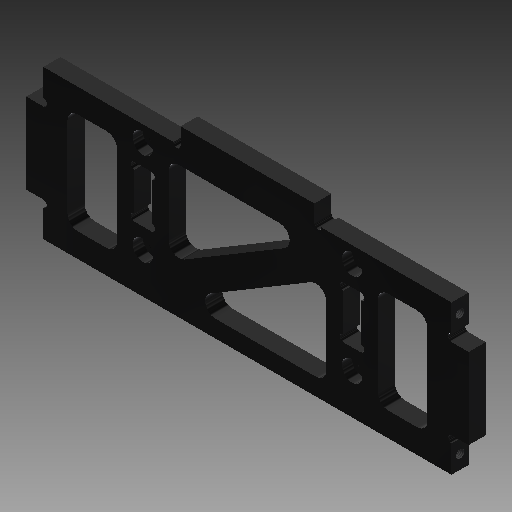
# Autodesk Inventor part: コックピット_サブフレーム_1_3
Saved by Autodesk Inventor 2018 (Build 220112000, 112)
## iProperties
Category: コックピット
Created: 2016-05-08
Part Number: コックピット_サブフレーム_1_3
Material: アセタール樹脂、黒
Document SubType Name: Modeling
Designer: hiroaki
Density: 1.425 g/cm^3
Appearance: 滑らか - 黒
Mass: 24.5118 g
Surface Area: 114.713 cm^2
Volume: 17.2013 cm^3
Author: hiroaki
Autodesk Inventor part; units mm, degrees
ref_plane "YZ Plane" through (0, 0, 0) normal (1, 0, 0) x (0, 1, 0)
ref_plane "XZ Plane" through (0, 0, 0) normal (0, 1, 0) x (-1, 0, 0)
ref_plane "XY Plane" through (0, 0, 0) normal (0, 0, 1) x (1, 0, 0)
sketch "スケッチ1" plane through (0, 0, 0) normal (0, 0, 1) x (1, 0, 0)
  line L0 (-59.5, -21.75) -> (59.5, -21.75) construction
  line L1 (59.5, -21.75) -> (59.5, 21.75) construction
  line L2 (59.5, 21.75) -> (-59.5, 21.75) construction
  line L3 (-59.5, 21.75) -> (-59.5, -21.75) construction
  line L4 (-59.5, -21.75) -> (59.5, 21.75) construction
  line L5 (59.5, -21.75) -> (-59.5, 21.75) construction
  line L6 (-54.5, -16.75) -> (54.5, -16.75) construction
  line L7 (54.5, -16.75) -> (54.5, 16.75) construction
  line L8 (54.5, 16.75) -> (-54.5, 16.75) construction
  line L9 (-54.5, 16.75) -> (-54.5, -16.75) construction
  line L10 (-54.5, -16.75) -> (54.5, 16.75) construction
  line L11 (54.5, -16.75) -> (-54.5, 16.75) construction
  line L12 (-33.05, 11.05) -> (-27.95, 11.05)
  line L13 (-27.95, 11.05) -> (-27.95, -4.05)
  line L14 (-27.95, -4.05) -> (-33.05, -4.05)
  line L15 (-33.05, -4.05) -> (-33.05, 11.05)
  line L16 (-28, 11) -> (-33, 11) construction
  line L17 (-33, 11) -> (-33, -4) construction
  line L18 (-33, -4) -> (-28, -4) construction
  line L19 (-28, -4) -> (-28, 11) construction
  line L20 (-30.5, 11) -> (-30.5, -4) construction
  line L21 (-33, 21) -> (-28, 21) construction
  line L22 (-28, 21) -> (-28, -14) construction
  line L23 (-28, -14) -> (-33, -14) construction
  line L24 (-33, -14) -> (-33, 21) construction
  circle A0 centre (-30.5, 17) radius 1.55
  circle A1 centre (-30.5, -10) radius 1.55
  circle A2 centre (-33.05, 10) radius 1.05
  circle A3 centre (-27.95, 10) radius 1.05
  circle A4 centre (-33.05, -3) radius 1.05
  circle A5 centre (-27.95, -3) radius 1.05
  line L25 (0, 0) -> (0, 16.75) construction
  line L26 (0, 0) -> (54.5, 0) construction
  circle A6 centre (30.5, 17) radius 1.55
  circle A7 centre (30.5, -10) radius 1.55
  circle A8 centre (27.95, 10) radius 1.05
  circle A9 centre (33.05, 10) radius 1.05
  circle A10 centre (27.95, -3) radius 1.05
  circle A11 centre (33.05, -3) radius 1.05
  line L27 (33.05, 11.05) -> (27.95, 11.05)
  line L28 (27.95, 11.05) -> (27.95, -4.05)
  line L29 (27.95, -4.05) -> (33.05, -4.05)
  line L30 (33.05, -4.05) -> (33.05, 11.05)
  line L31 (-59.5, 11.75) -> (-64.5, 11.75)
  line L32 (-64.5, 11.75) -> (-64.5, -11.75)
  line L33 (-64.5, -11.75) -> (-59.5, -11.75)
  line L34 (-59.5, 13.85) -> (-59.5, 21.75)
  line L35 (-59.5, 21.75) -> (-21.6, 21.75)
  line L36 (-19.5, 21.75) -> (-19.5, 26.75)
  line L37 (-19.5, 26.75) -> (19.5, 26.75)
  line L38 (19.5, 26.75) -> (19.5, 21.75)
  line L39 (21.6, 21.75) -> (59.5, 21.75)
  line L40 (59.5, 21.75) -> (59.5, 13.85)
  line L41 (59.5, 11.75) -> (64.5, 11.75)
  line L42 (64.5, 11.75) -> (64.5, -11.75)
  line L43 (64.5, -11.75) -> (59.5, -11.75)
  line L44 (-59.5, -13.85) -> (-59.5, -21.75)
  line L45 (-59.5, -21.75) -> (59.5, -21.75)
  line L46 (59.5, -21.75) -> (59.5, -13.85)
  arc A12 (-59.5, 11.75) -> (-59.5, 13.85) centre (-59.5, 12.8) ccw
  arc A13 (-59.5, -13.85) -> (-59.5, -11.75) centre (-59.5, -12.8) ccw
  line L47 (0, 0) -> (-54.5, 0) construction
  arc A14 (59.5, -11.75) -> (59.5, -13.85) centre (59.5, -12.8) ccw
  arc A15 (59.5, 13.85) -> (59.5, 11.75) centre (59.5, 12.8) ccw
  arc A16 (-21.6, 21.75) -> (-19.5, 21.75) centre (-20.55, 21.75) ccw
  arc A17 (19.5, 21.75) -> (21.6, 21.75) centre (20.55, 21.75) ccw
  line L48 (-56.8855, 19.3) -> (-54.5, 19.3) construction
  line L49 (-54.5, 19.3) -> (-54.5, 16.2) construction
  line L50 (-54.5, 16.2) -> (-56.8855, 16.2) construction
  line L51 (-56.8855, 16.2) -> (-56.8855, 19.3) construction
  line L52 (-54.5, 17.75) -> (-56.8855, 17.75) construction
  line L53 (-53.05, 22.7202) -> (-49.95, 22.7202) construction
  line L54 (-49.95, 22.7202) -> (-49.95, 16.75) construction
  line L55 (-49.95, 16.75) -> (-53.05, 16.75) construction
  line L56 (-53.05, 16.75) -> (-53.05, 22.7202) construction
  line L57 (-51.5, 22.7202) -> (-51.5, 16.75) construction
  point P0 (-30.5, -14)
  dimension "d10" = 2.1
  dimension "d0" = 33.5
  dimension "d1" = 5
  dimension "d2" = 109
  dimension "d3" = 5
  dimension "d4" = 0.05
  dimension "d5" = 35
  dimension "d6" = 27
  dimension "d7" = 5
  dimension "d11" = 33
  dimension "d12" = 3.1
  dimension "d13" = 1.05
  dimension "d14" = 5
  dimension "d15" = 4
  dimension "d16" = 3.1
  dimension "d17" = 10
  dimension "d18" = 5
  dimension "d19" = 8
  dimension "d20" = 5
  dimension "d21" = 40
  dimension "d22" = 5
  dimension "d50" = 4
  dimension "d51" = 10
  dimension "d52" = 17
  dimension "d53" = 10
  constraints: 114 end point, 19 perpendicular, 15 midpoint, 15 parallel, 14 centre point, 14 symmetric about line, 12 horizontal, 12 point on circle, 11 equal radius, 7 vertical alignment, 6 tangent, 5 point on line, 3 collinear, 3 vertical, 19 other
  measures "d0" distance of L6.end L7.end
  measures "d2" distance of L7.end L8.end
  measures "d3" distance between parallel lines of L3 L9
  measures "d4" distance between parallel lines of L13 L19
  measures "d5" distance of L21.end L22.end
  measures "d6" distance of A1.centre A0.centre
  measures "d7" distance of L21.start L21.end
  measures "d11" distance between parallel lines of L24 L25
  measures "d12" diameter of A0
  measures "d13" radius of A12
  measures "d14" distance between parallel lines of L32 L3
  measures "d16" distance of L48.end L49.end
  measures "d18" distance between parallel lines of L49 L3
  measures "d19" distance between parallel lines of L3 L57
  measures "d21" distance between parallel lines of L3 L36
  measures "d22" distance of L36.start L36.end
  measures "d50" distance from line of L21 A0.centre
  measures "d51" distance between parallel lines of L16 L21
  measures "d52" distance from line of L26 A0.centre
  measures "d53" distance between parallel lines of L18 L23
extrude "押し出し1" add sketch "スケッチ1" along normal blind 5
sketch "スケッチ2" plane through (0, 0, 5) normal (0, 0, 1) x (1, 0, 0)
  circle A0 centre (30.5, -10) radius 1.55 projected
  circle A1 centre (30.5, 17) radius 1.55 projected
  circle A2 centre (-30.5, -10) radius 1.55 projected
  circle A3 centre (-30.5, 17) radius 1.55 projected
  point P0 (0, 0)
  constraints: 4 coincident
hole "穴1" at (-30.5, 17, 5) at (-30.5, -10, 5) at (30.5, 17, 5) at (30.5, -10, 5) direction (0, 0, -1) diameter 6 depth 3
sketch "スケッチ3" plane through (59.5, -21.75, 0) normal (1, 0, 0) x (0, 0, -1)
  line L0 (0, 0) -> (-5, 0) projected
  line L1 (0, 43.5) -> (-5, 43.5) projected
  point P0 (0, 21.75)
  point P1 (-2.5, 4)
  point P2 (-2.5, 39.5)
  point P3 (-2.5, 0)
  dimension "d32" = 4
  dimension "d33" = 4
  constraints: 2 vertical alignment, 1 midpoint
  measures "d32" distance from line of L0 point (-2.5, 4)
  measures "d33" distance from line of L1 point (-2.5, 39.5)
hole "穴2" at (59.5, -17.75, 2.5) at (59.5, 17.75, 2.5) direction (-1, 0, 0) diameter 2.459 depth 2.5 thread size "M3x0.5" class "6H" standard "ISO Metric profile"
mirror "ミラー1" about plane through (0, 0, 0) normal (1, 0, 0) of "穴2"
sketch "スケッチ5" plane through (0, 0, 5) normal (0, 0, 1) x (1, 0, 0)
  line L0 (27.95, -1.95) -> (27.95, 8.95) projected
  line L1 (-33.05, -1.95) -> (-33.05, 8.95) projected
  line L2 (-27.95, 8.95) -> (-27.95, -1.95) projected
  line L3 (-59.5, -21.75) -> (59.5, -21.75) projected
  line L4 (19.5, 26.75) -> (-19.5, 26.75) projected
  line L5 (-21.6, 21.75) -> (-59.5, 21.75) projected
  line L6 (-59.5, 21.75) -> (-59.5, 13.85) projected
  line L7 (-52.5, 14.75) -> (-38, 14.75)
  line L8 (-38, 14.75) -> (-38, -14.75)
  line L9 (-38, -14.75) -> (-52.5, -14.75)
  line L10 (-52.5, -14.75) -> (-52.5, 14.75)
  line L11 (38, 14.75) -> (52.5, 14.75)
  line L12 (52.5, 14.75) -> (52.5, -14.75)
  line L13 (52.5, -14.75) -> (38, -14.75)
  line L14 (38, -14.75) -> (38, 14.75)
  line L15 (-23, 16.75) -> (-23, -9.0978)
  line L16 (-23, -9.0978) -> (20.2083, 16.75)
  line L17 (20.2083, 16.75) -> (-23, 16.75)
  line L18 (23, 9.0978) -> (23, -16.75)
  line L19 (23, -16.75) -> (-20.2083, -16.75)
  line L20 (-20.2083, -16.75) -> (23, 9.0978)
  line L21 (-33, 9.2736) -> (-28, 9.2736) construction
  line L22 (-28, 9.2736) -> (-28, -5.1442) construction
  line L23 (-28, -5.1442) -> (-33, -5.1442) construction
  line L24 (-33, -5.1442) -> (-33, 9.2736) construction
  line L25 (0, 0) -> (0, 26.75) construction
  line L26 (28, 10.3975) -> (29.3974, 10.3975) construction
  line L27 (29.3974, 10.3975) -> (29.3974, -4.5864) construction
  line L28 (29.3974, -4.5864) -> (28, -4.5864) construction
  line L29 (28, -4.5864) -> (28, 10.3975) construction
  line L30 (28, 16.75) -> (-28, -16.75) construction
  line L31 (-28, 16.75) -> (28, 16.75) construction
  line L32 (28, 16.75) -> (28, -16.75) construction
  line L33 (28, -16.75) -> (-28, -16.75) construction
  line L34 (-28, -16.75) -> (-28, 16.75) construction
  line L35 (59.5, 21.75) -> (21.6, 21.75) projected
  dimension "d54" = 7
  dimension "d55" = 7
  dimension "d56" = 7
  dimension "d57" = 0.05
  dimension "d58" = 5
  dimension "d59" = 0.05
  dimension "d60" = 5
  dimension "d62" = 5
  dimension "d63" = 0.05
  dimension "d64" = 8
  dimension "d68" = 5
  constraints: 56 end point, 14 parallel, 6 perpendicular, 5 horizontal, 4 collinear, 3 symmetric about line, 2 point on line, 1 midpoint, 1 vertical, 2 other
  measures "d54" distance between parallel lines of L6 L10
  measures "d55" distance between parallel lines of L5 L7
  measures "d56" distance between parallel lines of L3 L9
  measures "d57" distance between parallel lines of L1 L24
  measures "d58" distance between parallel lines of L8 L24
  measures "d59" distance between parallel lines of L2 L22
  measures "d60" distance between parallel lines of L15 L22
  measures "d62" distance between parallel lines of L3 L19
  measures "d63" distance between parallel lines of L0 L29
  measures "d64" distance between parallel lines of L20 L16
  measures "d68" distance between parallel lines of L35 L31
extrude "押し出し2" cut sketch "スケッチ5" against normal blind 10
fillet "フィレット1" radius 3 14 edges at (-38, 14.75, 2.5) (-52.5, 14.75, 2.5) (-52.5, -14.75, 2.5) (-38, -14.75, 2.5) (-23, -9.0978, 2.5) (-23, 16.75, 2.5) (20.2083, 16.75, 2.5) (23, 9.0978, 2.5) (-20.2083, -16.75, 2.5) (23, -16.75, 2.5) (38, -14.75, 2.5) (52.5, -14.75, 2.5) (52.5, 14.75, 2.5) (38, 14.75, 2.5)
equation "\"d20\" = d18"
equation "\"d53\" = d51"
equation "\"d32\" = d15"
equation "\"d33\" = d32"
equation "\"d56\" = d55"
equation "\"d59\" = d57"
equation "\"d60\" = d58"
